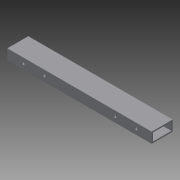
# Autodesk Inventor part: CatapultMotorSupport
Saved by Autodesk Inventor 2013 (Build 170138000, 138)
## iProperties
Created: 2014-01-18
Part Number: CatapultMotorSupport
Material: Generic
Document SubType Name: Modeling
Designer: 215152
Density: 1 g/cm^3
Author: 215152
Autodesk Inventor part; units mm, degrees
ref_plane "YZ Plane" through (0, 0, 0) normal (1, 0, 0) x (0, 1, 0)
ref_plane "XZ Plane" through (0, 0, 0) normal (0, 1, 0) x (-1, 0, 0)
ref_plane "XY Plane" through (0, 0, 0) normal (0, 0, 1) x (1, 0, 0)
sketch "Sketch1" plane through (0, 0, 0) normal (0, 1, 0) x (-1, 0, 0)
  line L0 (0, 0) -> (349.25, 0)
  line L1 (349.25, 0) -> (349.25, 50.8)
  line L2 (349.25, 50.8) -> (0, 50.8)
  line L3 (0, 50.8) -> (0, 0)
  dimension "d0" = 349.25
  dimension "d1" = 50.8
  constraints: 8 end point, 2 parallel, 1 horizontal, 1 perpendicular
  measures "d0" distance of L2.end L1.end
  measures "d1" distance of L1.end L0.end
extrude "Extrusion1" add sketch "Sketch1" along normal blind 25.4
sketch "Sketch2" plane through (0, 0, 50.8) normal (1, 0, 0) x (0, 0, -1)
  line L0 (0, 25.4) -> (3.175, 25.4)
  line L1 (3.175, 25.4) -> (3.175, 22.225)
  line L2 (3.175, 22.225) -> (0, 22.225)
  line L3 (0, 22.225) -> (0, 25.4)
  line L4 (3.175, 22.225) -> (47.625, 22.225)
  line L5 (47.625, 22.225) -> (47.625, 3.175)
  line L6 (47.625, 3.175) -> (3.175, 3.175)
  line L7 (3.175, 3.175) -> (3.175, 22.225)
  dimension "d4" = 3.175
  dimension "d5" = 3.175
  dimension "d6" = 44.45
  dimension "d7" = 19.05
  constraints: 16 end point, 4 parallel, 2 horizontal, 2 perpendicular
  measures "d4" distance of L1.end L2.end
  measures "d5" distance of L0.end L1.end
  measures "d6" distance of L5.end L6.end
  measures "d7" distance of L4.end L5.end
extrude "Extrusion2" cut sketch "Sketch2" against normal blind 508 contours L4 L5 L6 L7
sketch "Sketch3" plane through (-349.25, 0, 50.8) normal (0, 0, 1) x (1, 0, 0)
  line L0 (349.25, 0) -> (349.25, 25.4) projected
  line L1 (0, 0) -> (0, 25.4) projected
  line L2 (0, 12.7) -> (38.1, 12.7)
  line L3 (0, 12.7) -> (38.1, 12.7) construction
  line L4 (38.1, 12.7) -> (88.9, 12.7)
  circle A0 centre (88.9, 12.7) radius 3.175
  circle A1 centre (38.1, 12.7) radius 3.175
  line L5 (349.25, 12.7) -> (311.15, 12.7)
  line L6 (349.25, 12.7) -> (387.35, 12.7) construction
  line L7 (311.15, 12.7) -> (260.35, 12.7)
  line L8 (311.15, 12.7) -> (361.95, 12.7) construction
  circle A2 centre (260.35, 12.7) radius 3.175
  circle A3 centre (311.15, 12.7) radius 3.175
  dimension "d10" = 38.1
  dimension "d11" = 0
  dimension "d12" = 50.8
  dimension "d13" = 180
  dimension "d14" = 6.35
  dimension "d15" = 6.35
  dimension "d16" = 38.1
  dimension "d17" = 180
  dimension "d18" = 50.8
  dimension "d19" = 180
  dimension "d20" = 6.35
  dimension "d21" = 6.35
  constraints: 14 end point, 6 collinear, 4 centre point, 4 coincident, 3 horizontal, 2 midpoint, 1 perpendicular
  measures "d10" distance of L2.start L2.end
  measures "d11" distance between parallel lines of L2 L3
  measures "d12" distance of L2.end L4.end
  measures "d13" angle of L4 L2
  measures "d14" diameter of A0
  measures "d15" diameter of A1
  measures "d16" distance of L5.start L5.end
  measures "d17" angle of L5 L6
  measures "d18" distance of L5.end L7.end
  measures "d19" angle of L7 L8
  measures "d20" diameter of A2
  measures "d21" diameter of A3
extrude "Extrusion3" cut sketch "Sketch3" against normal blind 50.8
body "Solid1"
